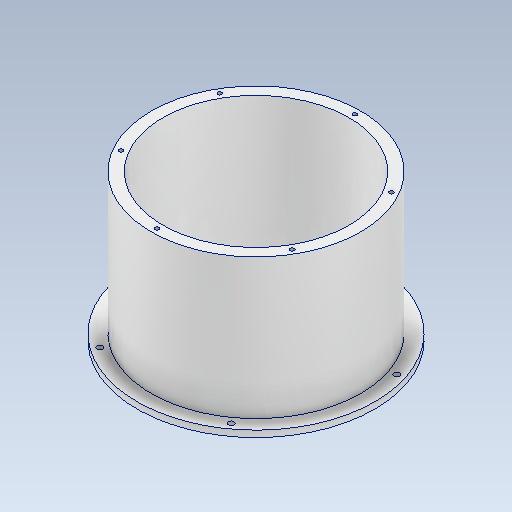
# Autodesk Inventor part: Base
Saved by Autodesk Inventor 2021 (Build 250183000, 183)
## iProperties
Created: 2020-05-10
Part Number: Base
Material: Aluminum 6061
Document SubType Name: Modeling
Designer: avi41
Density: 2.7 g/cm^3
Appearance: Aluminum - Flat
Author: avi41
Autodesk Inventor part; units mm, degrees
ref_plane "YZ Plane" through (0, 0, 0) normal (1, 0, 0) x (0, 1, 0)
ref_plane "XZ Plane" through (0, 0, 0) normal (0, 1, 0) x (-1, 0, 0)
ref_plane "XY Plane" through (0, 0, 0) normal (0, 0, 1) x (1, 0, 0)
sketch "Sketch2" plane through (0, 0, 0) normal (0, 0, 1) x (-1, 0, 0)
  line L0 (0, -22.8) -> (0, 136.8) construction
  line L1 (0, 114) -> (-92.5, 114)
  line L2 (-92.5, 114) -> (-92.5, 109)
  line L3 (-92.5, 109) -> (-81.5, 109)
  line L4 (-81.5, 109) -> (-81.5, 0)
  line L5 (-81.5, 0) -> (-72.5, 0)
  line L6 (-72.5, 0) -> (-72.5, 110)
  line L7 (-72.5, 110) -> (0, 110)
  line L8 (0, 114) -> (0, 110)
  line L9 (18.5, 0) -> (-111, 0) construction
  point P0 (0, 0)
  dimension "d4" = 5
  dimension "d5" = 11
  dimension "d6" = 9
  dimension "d8" = 110
  dimension "d9" = 4
  dimension "d38" = 81.5
  constraints: 16 end point, 7 perpendicular, 2 point on line, 1 collinear, 1 horizontal
  measures "d4" distance of L1.end L2.end
  measures "d5" distance between parallel lines of L2 L4
  measures "d6" distance between parallel lines of L4 L6
  measures "d8" distance between parallel lines of L7 L5
  measures "d9" distance between parallel lines of L1 L7
  measures "d38" distance between parallel lines of L0 L4
revolve "Revolution1" add sketch "Sketch2" angle 360 about axis through (0, 0, 0) along (0, -1, 0)
sketch "Sketch3" plane through (0, -109, 0) normal (0, 1, 0) x (1, 0, 0)
  line L0 (0, 129.5) -> (0, -129.5) construction
  line L1 (129.5, 0) -> (-129.5, 0) construction
  circle A0 centre (0, 0) radius 87 construction
  circle A1 centre (0, 0) radius 81.5 construction
  circle A2 centre (0, 0) radius 92.5 construction
  point P0 (0, 87)
  dimension "d11" = 5.5
  dimension "d12" = 5.5
  constraints: 1 coincident, 1 point on line, 1 vertical alignment, 2 other
hole "Hole1" at (0, -109, -87) direction (0, -1, 0) diameter 4.5 end through all clearance for "Flat Head Machine Screw" size "M4" standard "Ansi Metric M Profile"
pattern_circular "Circular Pattern1" count 5 over 360 about axis through (0, -10, 0) along (0, 1, 0) of "Hole1"
sketch "Sketch5" plane through (0, 0, 0) normal (0, 1, 0) x (1, 0, 0)
  line L0 (0, 129.5) -> (0, -129.5) construction
  line L1 (129.5, 0) -> (-129.5, 0) construction
  circle A0 centre (0, 0) radius 77 construction
  circle A1 centre (0, 0) radius 72.5 construction
  circle A2 centre (0, 0) radius 81.5 construction
  point P0 (0, 77)
  point P1 (-66.684, 38.5)
  point P2 (-66.684, -38.5)
  point P3 (0, -77)
  point P4 (66.684, -38.5)
  point P5 (66.684, 38.5)
  dimension "d39" = 4.5
  dimension "d40" = 4.5
  dimension "d43" = 360
  constraints: 3 coincident, 1 point on line, 1 vertical alignment, 13 other
hole "Hole2" at (0, 0, -77) at (-66.684, 0, -38.5) at (-66.684, 0, 38.5) at (0, 0, 77) at (66.684, 0, 38.5) at (66.684, 0, -38.5) direction (0, -1, 0) diameter 3.242 depth 13 tip angle 118 thread size "M4x0.7" class "6H" standard "ANSI Metric M Profile"
equation "\"d11\" = d12"
equation "\"d39\" = d40"
body "Solid2"
